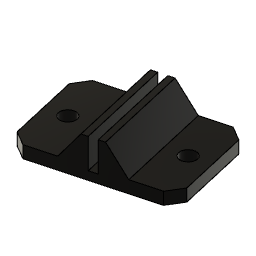
Mount stop (Autodesk Fusion 360 design; units mm, degrees)
Autodesk Fusion 360 part; units mm, degrees
box "BoitePrimitive1" add length 40 width 27.5 height 5 placed x (0, 0, 1) y (1, 0, 0) z (0, 1, 0) at (-32.5, 0, 0) makes body 1
sketch "Esquisse2" plane through (0, 5, 0) normal (0, 1, 0) x (-1, 0, 0)
  line L0 (32.5, 40) -> (5, 40)
  line L1 (5, 40) -> (5, 0)
  line L2 (5, 0) -> (32.5, 0)
  line L3 (32.5, 0) -> (32.5, 40)
  line L4 (13.5, 0) -> (13.5, 40) construction
  circle A0 centre (13.5, 20) radius 3.3
  line L5 (22, 0) -> (22, 40)
  line L6 (5, 20) -> (22, 20) construction
  dimension "d9" = 8.5
  dimension "d14" = 6.6
  dimension "d23" = 17
  constraint coincident L2 L4.start
  constraint coincident L0 L4.end
  constraint perpendicular L0 L4
  constraint coincident L4 A0.centre
  constraint coincident L2 L5.start
  constraint coincident L0 L5.end
  constraint perpendicular L0 L5
  constraint midpoint L1 L6.start
  constraint midpoint L5 L6.end
  constraint midpoint L4 A0.centre
  measures "d9" distance of L1 L4
  measures "d14" diameter of A0
  measures "d23" distance of L1 L5
extrude "Extrusion2" cut sketch "Esquisse2" against normal through all contours A0 bodies 1
extrude "Extrusion3" add sketch "Esquisse2" along normal blind 10.6 contours L0 L2 L3 L5 bodies 1
chamfer "Chanfrein2" distance 8 distance2 10.6 1 edges at (-22, 15.6, 20) measured on face at (-25.5, 15.6, 13.3333) on bodies 1
chamfer "Chanfrein3" distance 5 angle 45 2 edges at (-5, 2.5, 40) (-5, 2.5, 0) on bodies 1
ref_plane "Plan de construction1" through (-34.25, 7.8, 20) normal (-1, 0, 0) x (0, -1, 0)
mirror "Symétrie miroir1" about plane through (-34.25, 7.8, 20) normal (-1, 0, 0) of bodies 1 makes body 2
sketch "Esquisse5" plane through (-32.5, 0, 0) normal (-1, 0, 0) x (0, 0, 1)
  line L0 (0, 15.6) -> (0, 0)
  line L1 (0, 0) -> (40, 0)
  line L2 (40, 0) -> (40, 15.6)
  line L3 (40, 15.6) -> (0, 15.6)
  line L4 (0, 3.4) -> (40, 3.4)
  dimension "d34" = 3.4
  constraint coincident L0 L4.start
  constraint coincident L2 L4.end
  constraint perpendicular L2 L4
  measures "d34" distance of L1 L4
extrude "Extrusion4" add sketch "Esquisse5" along normal up to surface (3.5 mm away) contours L0 L1 L2 L4 bodies 1 2
equation "d1 = long"
equation "d2 = larg"
equation "d3 = ep"
equation "vis_diam = 6 mm"
equation "vis_jeu = 0.6 mm"
equation "d14 = vis_diam + vis_jeu"
equation "long = 40 mm"
equation "larg = 27.5 mm"
equation "ep = 5 mm"
equation "haut = 15.6 mm"
equation "d24 = haut - ep"
equation "d27 = haut - ep"
equation "écartement = 3.3 mm"
equation "écartement_jeu = 0.2 mm"
equation "d30 = ( écartement + écartement_jeu ) / 2"
equation "ep2 = 3.4 mm"
equation "d34 = ep2"
named bodies: "Mount stop"
